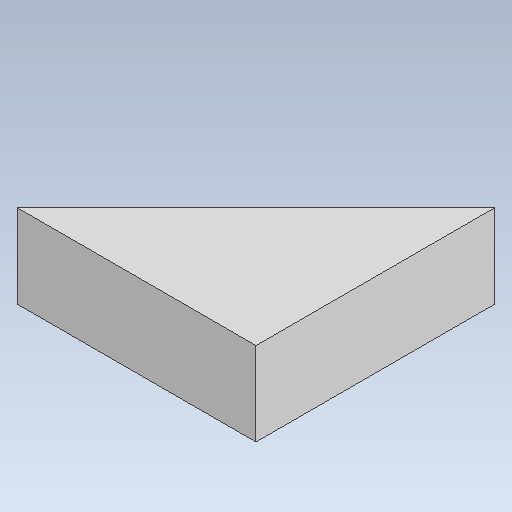
# Autodesk Inventor part: BonsaiFeet
Saved by Autodesk Inventor 2020 (Build 240168000, 168)
## iProperties
Created: 2020-05-10
Part Number: BonsaiFeet
Material: Generic
Document SubType Name: Modeling
Designer: user
Density: 1 g/cm^3
Appearance: Default
Author: user
Autodesk Inventor part; units mm, degrees
ref_plane "YZ Plane" through (0, 0, 0) normal (1, 0, 0) x (0, 1, 0)
ref_plane "XZ Plane" through (0, 0, 0) normal (0, 1, 0) x (-1, 0, 0)
ref_plane "XY Plane" through (0, 0, 0) normal (0, 0, 1) x (1, 0, 0)
sketch "Sketch1" plane through (0, 0, 0) normal (0, 1, 0) x (-1, 0, 0)
  line L0 (5.4891, 8.0164) -> (-14.5109, 8.0164)
  line L1 (-14.5109, 8.0164) -> (-14.5109, -11.9836)
  line L2 (-14.5109, -11.9836) -> (5.4891, 8.0164)
  point P0 (0, 0)
  dimension "d6" = 90
  dimension "d7" = 45
  dimension "d8" = 20
  dimension "d9" = 20
  constraints: 6 end point, 1 horizontal, 1 perpendicular
  measures "d6" angle of L0 L1
  measures "d7" angle of L2 L1
  measures "d8" distance of L0.end L1.end
  measures "d9" distance from line of L1 L0.start
extrude "Extrusion1" add sketch "Sketch1" along normal blind 7
body "Solid1"
